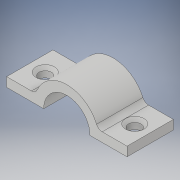
# Autodesk Inventor part: CableWallMount
Saved by Autodesk Inventor 2018 (Build 220112000, 112)
## iProperties
Created: 2021-02-03
Part Number: CableWallMount
Material: Generic
Document SubType Name: Modeling
Designer: dangl
Density: 1 g/cm^3
Appearance: Default
Author: dangl
Autodesk Inventor part; units mm, degrees
ref_plane "YZ Plane" through (0, 0, 0) normal (1, 0, 0) x (0, 1, 0)
ref_plane "XZ Plane" through (0, 0, 0) normal (0, 1, 0) x (-1, 0, 0)
ref_plane "XY Plane" through (0, 0, 0) normal (0, 0, 1) x (1, 0, 0)
sketch "Sketch1" plane through (0, 0, 0) normal (0, 0, 1) x (1, 0, 0)
  arc A0 (0, 7.5) -> (-7.5, 0) centre (0, 0) ccw
  line L0 (-7.5, 0) -> (-19.5, 0)
  line L1 (-19.5, 0) -> (-19.5, 3)
  arc A1 (0, 10.5) -> (-9.6234, 4.2) centre (0, 0) ccw
  line L2 (-19.5, 3) -> (-11.4564, 3)
  line L3 (0, 10.5) -> (0, 7.5)
  arc A2 (-11.4564, 3) -> (-9.6234, 4.2) centre (-11.4564, 5) ccw
  point P0 (-10.0623, 3)
  dimension "d0" = 15
  dimension "d1" = 12
  dimension "d2" = 3
  dimension "d3" = 3
  dimension "d4" = 2
  constraints: 8 end point, 7 point on circle, 3 centre point, 2 horizontal, 2 tangent, 2 vertical, 1 coincident, 1 point on line
  measures "d0" diameter of A0
  measures "d1" distance of L0.start L0.end
  measures "d2" distance of L0.end L1.end
  measures "d3" radial gap between concentric circles of A0 A1
  measures "d4" radius of A2
extrude "Extrusion1" add sketch "Sketch1" along normal mid plane 15
sketch "Sketch2" plane through (-19.5, 3, 7.5) normal (0, 1, 0) x (1, 0, 0)
  line L0 (-3.9, 7.5) -> (23.4, 7.5) projected
  circle A0 centre (5, 7.5) radius 2
  line L1 (0, 15) -> (0, 0) projected
  point P0 (19.5, 7.5)
  dimension "d7" = 4
  dimension "d8" = 5
  constraints: 1 centre point, 1 point on line
  measures "d7" diameter of A0
  measures "d8" distance from line of L1 A0.centre
extrude "Extrusion2" cut sketch "Sketch2" against normal blind 15
chamfer "Chamfer1" distance 1 angle 45 1 edges at (-16.5, 3, 0)
mirror "Mirror1" about plane through (0, 7.5, 0) normal (1, 0, 0) of "Extrusion1", "Extrusion2", "Chamfer1"
body "Solid1"
